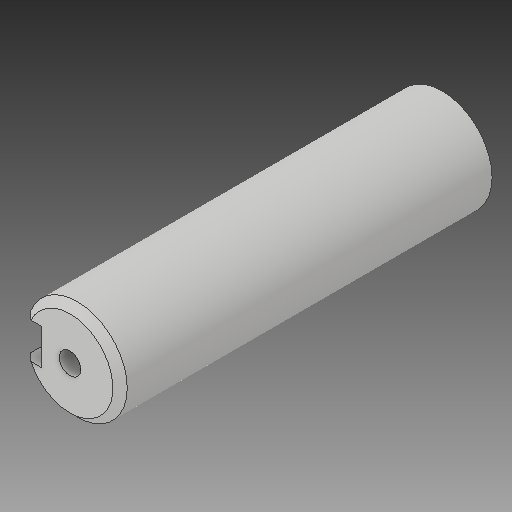
# Autodesk Inventor part: Shaft
Saved by Autodesk Inventor 2018 (Build 220112000, 112)
## iProperties
Created: 2017-05-16
Part Number: Shaft
Material: Generic
Document SubType Name: Modeling
Designer: M220404
Density: 1 g/cm^3
Appearance: Default
Author: M220404
Autodesk Inventor part; units mm, degrees
ref_plane "XZ Plane" through (0, 0, 0) normal (0, 1, 0) x (-1, 0, 0)
ref_plane "XY Plane" through (0, 0, 0) normal (0, 0, 1) x (1, 0, 0)
sketch "Sketch1" plane through (0, 0, 0) normal (0, 0, 1) x (1, 0, 0)
  circle A0 centre (0, 0) radius 7
  dimension "d0" = 14
  constraints: 1 centre point, 1 coincident
  measures "d0" diameter of A0
extrude "Extrusion1" add sketch "Sketch1" along normal blind 52
hole "Hole1" at (0, 0, 52) direction (0, 0, -1) diameter 3 depth 13
ref_plane "Work Plane1" through (-7, 0, 0) normal (1, 0, 0) x (0, 1, 0)
sketch "Sketch2" plane through (-7, 0, 0) normal (1, 0, 0) x (0, 1, 0)
  line L0 (-2.5, 29.5) -> (-2.5, 52)
  line L1 (-2.5, 52) -> (2.5, 52)
  line L2 (2.5, 52) -> (2.5, 29.5)
  line L3 (7, 52) -> (-7, 52) projected
  line L4 (7, 52) -> (-7, 52) projected
  line L5 (-7, 0) -> (7, 0) projected
  line L6 (7, 0) -> (7, 52) projected
  line L7 (-7, 0) -> (-7, 52) projected
  arc A0 (-2.5, 29.5) -> (2.5, 29.5) centre (0, 29.5) ccw
  point P0 (0, 0)
  point P1 (0, 27)
  dimension "d12" = 5
  dimension "d14" = 0
  constraints: 6 end point, 3 point on circle, 1 centre point, 1 parallel, 1 tangent
  measures "d12" distance of L0.end L1.end
  measures "d14" distance between parallel lines of L3 L1
extrude "Extrusion2" cut sketch "Sketch2" along normal blind 3 contours L0 L1 L2 A0
chamfer "Chamfer1" distance 1 angle 45 2 edges at (1.2711, -6.8836, 52) (1.2711, 6.8836, 52)
body "Solid1"
